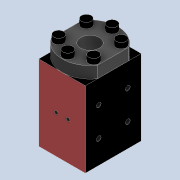
# Autodesk Inventor part: Z Axis Statonary Block
Saved by Autodesk Inventor 2022 (Build 260153000, 153)
## iProperties
Created: 2021-10-24
Part Number: Z Axis Statonary Block
Material: Generic
Document SubType Name: Modeling
Designer: Coy
Density: 1 g/cm^3
Appearance: Anodized - Black
Author: Coy
Autodesk Inventor part; units mm, degrees
ref_plane "YZ Plane" through (0, 0, 0) normal (1, 0, 0) x (0, 1, 0)
ref_plane "XZ Plane" through (0, 0, 0) normal (0, 1, 0) x (-1, 0, 0)
ref_plane "XY Plane" through (0, 0, 0) normal (0, 0, 1) x (1, 0, 0)
sketch "Sketch1" plane through (0, 0, 0) normal (1, 0, 0) x (0, 1, 0)
  line L0 (0, 0) -> (65, 0)
  line L1 (65, 0) -> (65, 48)
  line L2 (65, 48) -> (0, 48)
  line L3 (0, 48) -> (0, 0)
  dimension "d0" = 65
  dimension "d1" = 48
  constraints: 8 end point, 2 parallel, 1 horizontal, 1 perpendicular
  measures "d0" distance of L1.end L2.end
  measures "d1" distance of L0.end L1.end
extrude "Extrusion1" add sketch "Sketch1" against normal blind 40
sketch "Sketch2" plane through (0, 0, 0) normal (1, 0, 0) x (0, 0, -1)
  line L0 (-36.5, 45) -> (-11.5, 45) construction
  line L1 (-11.5, 45) -> (-11.5, 20) construction
  line L2 (-11.5, 20) -> (-36.5, 20) construction
  line L3 (-36.5, 20) -> (-36.5, 45) construction
  line L4 (-36.5, 45) -> (-36.5, 65) construction
  line L5 (-48, 65) -> (0, 65) construction
  line L6 (-36.5, 45) -> (-48, 45) construction
  line L7 (-48, 0) -> (-48, 65) construction
  line L8 (-11.5, 20) -> (-11.5, 0) construction
  line L9 (0, 0) -> (-48, 0) construction
  line L10 (-11.5, 20) -> (0, 20) construction
  circle A0 centre (-36.5, 45) radius 2
  circle A1 centre (-11.5, 45) radius 2
  circle A2 centre (-11.5, 20) radius 2
  circle A3 centre (-36.5, 20) radius 2
  line L11 (0, 0) -> (0, 65) projected
  dimension "d4" = 25
  dimension "d5" = 25
  dimension "d6" = 4
  dimension "d7" = 4
  dimension "d8" = 4
  dimension "d9" = 4
  constraints: 16 end point, 4 centre point, 4 coincident, 4 parallel, 4 point on line, 3 perpendicular, 2 horizontal, 1 vertical
  measures "d4" distance of L0.start L0.end
  measures "d5" distance of L0.end L1.end
  measures "d6" diameter of A0
  measures "d7" diameter of A1
  measures "d8" diameter of A2
  measures "d9" diameter of A3
extrude "Extrusion2" cut sketch "Sketch2" against normal blind 8
sketch "Sketch3" plane through (0, 0, 48) normal (0, 0, 1) x (1, 0, 0)
  line L0 (0, 65) -> (0, 0) construction
  line L1 (0, 32.5) -> (-40, 32.5) construction
  line L2 (-40, 0) -> (-40, 65) construction
  line L3 (-25, 32.5) -> (-15, 32.5) construction
  circle A0 centre (-25, 32.5) radius 1.5
  circle A1 centre (-15, 32.5) radius 1.5
  dimension "d12" = 10
  dimension "d13" = 15
  dimension "d14" = 3
  dimension "d15" = 3
  constraints: 4 end point, 2 centre point, 2 coincident, 2 midpoint, 2 point on line
  measures "d12" distance of L3.start L3.end
  measures "d13" distance of L1.start L3.end
  measures "d14" diameter of A0
  measures "d15" diameter of A1
extrude "Extrusion3" cut sketch "Sketch3" against normal blind 6
sketch "Sketch4" plane through (0, 0, 0) normal (0, 0, -1) x (-1, 0, 0)
  circle A0 centre (25, 32.5) radius 1.5 projected
  circle A1 centre (15, 32.5) radius 1.5 projected
  point P0 (0, 0)
extrude "Extrusion4" cut sketch "Sketch4" against normal blind 6
thread "Thread1" size "M3x0.5" class "6H" standard "ANSI Metric M Profile" full length
thread "Thread2" size "M3x0.5" class "6H" standard "ANSI Metric M Profile" full length
thread "Thread3" size "M4x0.7" class "6H" standard "ANSI Metric M Profile" full length
thread "Thread4" size "M4x0.7" class "6H" standard "ANSI Metric M Profile" full length
thread "Thread5" size "M4x0.7" class "6H" standard "ANSI Metric M Profile" full length
thread "Thread6" size "M4x0.7" class "6H" standard "ANSI Metric M Profile" full length
thread "Thread7" size "M3x0.5" class "6H" standard "ANSI Metric M Profile" full length
thread "Thread8" size "M3x0.5" class "6H" standard "ANSI Metric M Profile" full length
sketch "Sketch5" plane through (0, 65, 48) normal (0, 1, 0) x (1, 0, 0)
  line L0 (-40, 48) -> (-40, 0) projected
  line L1 (-40, 10.5) -> (-40, 37.5)
  line L2 (0, 0) -> (0, 48) projected
  line L3 (0, 10.5) -> (0, 37.5)
  line L4 (0, 38.5) -> (-8, 38.5) projected
  arc A0 (-40, 10.5) -> (0, 10.5) centre (-20, 24.2976) ccw
  arc A1 (0, 37.5) -> (-40, 37.5) centre (-20, 23.7024) ccw
  line L5 (-0.01, 10.5031) -> (-0.01, 37.4969)
  arc A2 (-0.01, 37.4969) -> (-39.99, 37.4969) centre (-20, 23.7024) ccw
  line L6 (-39.99, 37.4969) -> (-39.99, 10.5031)
  arc A3 (-39.99, 10.5031) -> (-0.01, 10.5031) centre (-20, 24.2976) ccw
  line L7 (-39.99, 24) -> (-0.01, 24) construction
  circle A4 centre (-20, 24) radius 8
  dimension "d36" = 27
  dimension "d37" = 10.5
  dimension "d38" = 0.01
  dimension "d39" = 16
  constraints: 10 end point, 8 point on circle, 5 centre point, 3 midpoint, 3 point on line, 1 perpendicular, 3 other
  measures "d36" distance of L1.start L1.end
  measures "d37" distance of L0.end L1.start
  measures "d38" radial gap between concentric circles of A0 A3
  measures "d39" diameter of A4
extrude "Extrusion5" add sketch "Sketch5" along normal blind 10 contours A2 L5 A3 L6
sketch "Sketch6" plane through (0, 75, 48) normal (0, 1, 0) x (1, 0, 0)
  arc A0 (-0.01, 37.4969) -> (-39.99, 37.4969) centre (-20, 23.7024) ccw projected
  line L0 (-39.99, 37.4969) -> (-39.99, 10.5031) projected
  arc A1 (-39.99, 10.5031) -> (-0.01, 10.5031) centre (-20, 24.2976) ccw projected
  line L1 (-0.01, 10.5031) -> (-0.01, 37.4969) projected
  circle A2 centre (-20, 24) radius 8 projected
  arc A3 (-5.01, 35.8396) -> (-34.99, 35.8396) centre (-20, 23.7024) ccw construction
  line L2 (-5.01, 35.8396) -> (-5.01, 12.1604) construction
  arc A4 (-34.99, 12.1604) -> (-5.01, 12.1604) centre (-20, 24.2976) ccw construction
  line L3 (-34.99, 12.1604) -> (-34.99, 35.8396) construction
  circle A5 centre (-34.99, 35.8396) radius 4.25
  circle A6 centre (-20, 42.99) radius 4.25
  circle A7 centre (-5.01, 35.8396) radius 4.25
  circle A8 centre (-5.01, 12.1604) radius 4.25
  circle A9 centre (-20, 5.01) radius 4.25
  circle A10 centre (-34.99, 12.1604) radius 4.25
  point P0 (0, 48)
  dimension "d42" = 5
  dimension "d43" = 8.5
  dimension "d44" = 8.5
  dimension "d45" = 8.5
  dimension "d46" = 8.5
  dimension "d47" = 8.5
  dimension "d48" = 8.5
  constraints: 8 centre point, 6 point on circle, 4 coincident, 4 end point, 3 other
  measures "d42" radial gap between concentric circles of A0 A3
  measures "d43" diameter of A5
  measures "d44" diameter of A6
  measures "d45" diameter of A7
  measures "d46" diameter of A8
  measures "d47" diameter of A9
  measures "d48" diameter of A10
extrude "Extrusion6" add sketch "Sketch6" along normal blind 4.75 contours A5 | A6 | A7 | A8 | A9 | A10
sketch "Sketch7" plane through (-20, 65, 24) normal (0, 1, 0) x (1, 0, 0)
  circle A0 centre (0, 0) radius 8 projected
  point P0 (20, 24)
extrude "Extrusion7" cut sketch "Sketch7" against normal up to next
equation "\"d7\" = d6"
equation "\"d8\" = d6"
equation "\"d9\" = d6"
equation "\"d15\" = d14"
equation "\"d44\" = d43"
equation "\"d45\" = d43"
equation "\"d46\" = d43"
equation "\"d47\" = d43"
equation "\"d48\" = d43"
body "Solid1"
